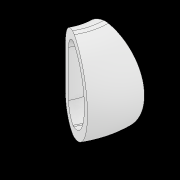
# Autodesk Inventor part: L_Notch1-Wedge
Saved by Autodesk Inventor 2021 (Build 250183000, 183)
## iProperties
Created: 2020-11-13
Part Number: L_Notch1-Wedge
Material: UHMW, White
Document SubType Name: Modeling
Designer: Eli Mattingly
Density: 0.94 g/cm^3
Appearance: Smooth - White
Author: Eli Mattingly
Autodesk Inventor part; units mm, degrees
ref_plane "Work Plane1" through (-7, 0, -29.5697) normal (1, 0, 0) x (0, 0, -1)
ref_plane "YZ Plane" through (0, 0, 0) normal (1, 0, 0) x (0, 1, 0)
ref_plane "XZ Plane" through (0, 0, 0) normal (0, 1, 0) x (-1, 0, 0)
sketch "Sketch1" plane through (0, 0, 0) normal (0, 0, 1) x (1, 0, 0)
  line L0 (0, 0) -> (0, 16.1) construction
  line L1 (10.73, 8.24) -> (10.73, -8.24)
  line L2 (18.59, 16.1) -> (18.59, -16.1) construction
  arc A0 (17.6161, 16.0394) -> (10.73, 8.24) centre (18.59, 8.24) ccw
  arc A1 (10.73, -8.24) -> (17.6161, -16.0394) centre (18.59, -8.24) ccw
  arc A2 (19.284, -15.9668) -> (19.284, 15.9668) centre (15.8602, 0) ccw
  line L3 (0, 0) -> (51.4073, 0)
  arc A3 (19.284, 15.9668) -> (17.6161, 16.0394) centre (18.2356, 11.078) ccw
  arc A4 (17.6161, -16.0394) -> (19.284, -15.9668) centre (18.2356, -11.078) ccw
  arc A5 (18.655, 13.0335) -> (17.9878, 13.0626) centre (18.2356, 11.078) ccw
  arc A6 (17.9878, 13.0626) -> (13.73, 8.24) centre (18.59, 8.24) ccw
  line L4 (13.73, 8.24) -> (13.73, -8.24)
  arc A7 (13.73, -8.24) -> (17.9878, -13.0626) centre (18.59, -8.24) ccw
  arc A8 (17.9878, -13.0626) -> (18.655, -13.0335) centre (18.2356, -11.078) ccw
  arc A9 (18.655, -13.0335) -> (18.655, 13.0335) centre (15.8602, 0) ccw
  point P0 (10.73, 0)
  point P1 (32.19, 0)
  point P2 (18.59, 0)
  dimension "MaxHeight" = 16.1
  dimension "FlatHeightx2" = 16.48
  dimension "ID" = 21.46
  dimension "OD" = 64.38
  dimension "d5" = 32.2
  dimension "RadAtPeak" = 18.59
  dimension "d90" = 5
  dimension "d97" = 3
  constraints: 25 point on circle, 10 centre point, 10 end point, 5 tangent, 3 horizontal alignment, 3 vertical, 2 line through centre, 2 midpoint, 1 equal radius, 1 horizontal, 5 other
  measures "MaxHeight" distance of L0.start L0.end
  measures "FlatHeightx2" distance of L1.start L1.end
  measures "ID" diameter of L1 L0
  measures "OD" diameter of point (32.19, 0) L0
  measures "d5" distance of L2.start L2.end
  measures "RadAtPeak" distance from line of L0.start L2
  measures "d90" radius of A3
  measures "d97" radial gap between concentric circles of A2 A9
revolve "Revolution1" add sketch "Sketch1" angle 30 about axis through (0, 0, 0) along (0, -1, 0) contours A0 A3 A2 L3 A9 A5 A6 L4 L1 | L3 L4 A7 A8 A9 A2 A4 A1 L1
sketch "Sketch13" plane through (10.73, -8.24, 0) normal (0, 0, -1) x (-1, 0, 0)
  arc A0 (0, 16.48) -> (-6.8861, 24.2794) centre (-7.86, 16.48) ccw projected
  arc A1 (-6.8861, 24.2794) -> (-8.554, 24.2068) centre (-7.5056, 19.318) ccw projected
  arc A2 (-8.554, 24.2068) -> (-8.6304, 24.1903) centre (-5.1302, 8.24) ccw projected
  arc A3 (-8.554, -7.7268) -> (-6.8861, -7.7994) centre (-7.5056, -2.838) ccw projected
  arc A4 (-6.8861, -7.7994) -> (0, 0) centre (-7.86, 0) ccw projected
  line L0 (0, 16.48) -> (0, 0) projected
  line L1 (-7.86, 0) -> (3, 0)
  line L2 (3, 0) -> (3, 16.48)
  line L3 (3, 16.48) -> (-7.86, 16.48)
  line L4 (-7.86, 16.48) -> (-7.86, 0)
  arc A5 (-8.6304, 24.1903) -> (-8.6304, -7.7103) centre (-5.1302, 8.24) ccw projected
  point P0 (10.73, 8.24)
  point P1 (-4.6967, 8.3392)
  dimension "d93" = 3
  constraints: 8 end point, 2 parallel, 1 horizontal, 1 horizontal alignment, 1 perpendicular, 3 other
  measures "d93" distance between parallel lines of L0 L2
sketch "Sketch7" plane through (0, 0, 0) normal (0, 1, 0) x (-1, 0, 0)
  circle A0 centre (0, 0) radius 198.9616
  constraints: 1 centre point, 1 coincident
sketch "Sketch8" plane through (0, 0, 0) normal (1, 0, 0) x (0, 1, 0)
  circle A0 centre (0, 0) radius 159.0195
  constraints: 1 centre point, 1 coincident
sketch "Sketch9" plane through (0, 0, 0) normal (1, 0, 0) x (0, 0, -1)
  line L0 (74, 0) -> (35, 0) projected
  point P0 (0, 0)
  point P1 (-52.5, 0)
  point P2 (0, 0)
  point P3 (52.5, 0)
  dimension "d88" = 105
  dimension "d89" = 52.5
  constraints: 1 point on line
  measures "d88" distance of point (52.5, 0) point (-52.5, 0)
  measures "d89" distance of point (52.5, 0) point (0, 0)
sketch "Sketch11" plane through (0, 0, 0) normal (1, 0, 0) x (0, 0, -1)
  arc A0 (-35, 25.9107) -> (-42.6927, 34.8921) centre (-44.0893, 25.9107) ccw projected
  line L0 (-35, 25.9107) -> (-35, 0) projected
  line L1 (-35, 0) -> (35, 0) projected
  arc A1 (-50.0415, 0) -> (-54.9585, 0) centre (-52.5, 0) ccw projected
  arc A2 (-50.0415, 0) -> (-54.9585, 0) centre (-37.5, 0) ccw projected
  arc A3 (-39.8678, 39.0634) -> (-73, 0) centre (-33.4058, 0) ccw
  arc A4 (-29.5697, 27.789) -> (-36.4391, 38.3935) centre (-44.0893, 25.9107) ccw
  line L2 (-29.5697, 27.789) -> (-29.5697, 0)
  line L3 (-35, 0) -> (35, 0) projected
  line L4 (-73, 0) -> (-29.5697, 0)
  arc A5 (-36.4391, 38.3935) -> (-39.8678, 39.0634) centre (-39.0518, 34.1304) ccw
  point P0 (0, 0)
  point P1 (-35, 0)
  point P2 (-29.5697, 0)
  point P3 (-54.9585, 0)
  point P4 (-50.0415, 0)
  dimension "d91" = 5
  constraints: 6 point on circle, 4 end point, 3 centre point, 2 tangent, 1 horizontal, 1 point on line, 1 other
  measures "d91" radius of A5
sketch "Sketch6" plane through (0.6222, 0, 0.3592) normal (-0.5, 0, 0.866) x (0, 1, 0)
  line L0 (-8.24, -10.0116) -> (8.24, -10.0116) projected
  arc A0 (-15.9668, -18.5655) -> (15.9668, -18.5655) centre (0, -15.1418) ccw projected
  arc A1 (-17.2892, -21.2298) -> (17.2892, -21.2298) centre (0, -15.1418) ccw
  line L1 (15.9668, -18.5655) -> (15.4028, -18.5655)
  arc A2 (17.2892, -21.2298) -> (15.4028, -18.5655) centre (15.4028, -20.5655) ccw
  line L2 (-15.4028, -18.5655) -> (-15.9668, -18.5655)
  arc A3 (-15.4028, -18.5655) -> (-17.2892, -21.2298) centre (-15.4028, -20.5655) ccw
  line L3 (-25.2101, 0.7184) -> (25.2101, 0.7184) projected
  point P0 (0, 0.7184)
  point P1 (-18.0072, -18.5655)
  point P2 (18.0072, -18.5655)
  point P3 (15.9503, -18.6419)
  point P4 (-15.9503, -18.6419)
  dimension "d47" = 2
  dimension "d48" = 2
  dimension "d49" = 2
  constraints: 8 point on circle, 4 end point, 4 tangent, 3 centre point, 2 point on line, 1 horizontal
  measures "d47" radial gap between concentric circles of A0 A1
  measures "d48" radius of A2
  measures "d49" radius of A3
equation "\"d5\" = 2 * MaxHeight"
equation "\"d63_Copy\" = 35"
body "Solid1"
